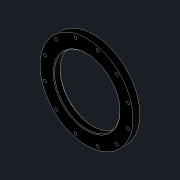
# Autodesk Inventor part: unit-j2-base2
Saved by Autodesk Inventor 2022 (Build 260153000, 153)
## iProperties
Created: 2021-07-12
Part Number: unit-j2-base2
Material: ABS プラスチック
Document SubType Name: Modeling
Designer: yuta0
Density: 1.06 g/cm^3
Appearance: 滑らか - 黒
Mass: 58.1208 g
Surface Area: 198.021 cm^2
Volume: 54.831 cm^3
購入先: 印刷
在庫数: 0.0
Author: yuta0
Autodesk Inventor part; units mm, degrees
ref_plane "YZ Plane" through (0, 0, 0) normal (1, 0, 0) x (0, 1, 0)
ref_plane "XZ Plane" through (0, 0, 0) normal (0, 1, 0) x (-1, 0, 0)
ref_plane "XY Plane" through (0, 0, 0) normal (0, 0, 1) x (1, 0, 0)
sketch "スケッチ1" plane through (0, 0, 0) normal (0, 0, 1) x (1, 0, 0)
  circle A0 centre (0, 0) radius 47.6
  circle A1 centre (0, 0) radius 67.5
  dimension "d0" = 95.2
  dimension "d1" = 135
  constraints: 2 centre point, 2 coincident
  measures "d0" diameter of A0
  measures "d1" diameter of A1
extrude "押し出し1" add sketch "スケッチ1" along normal blind 10
sketch "スケッチ2" plane through (0, 0, 10) normal (0, 0, 1) x (1, 0, 0)
  circle A0 centre (0, 0) radius 62.5
  point P0 (16.1762, 60.3704)
  point P1 (-16.1762, 60.3704)
  point P2 (-44.1942, 44.1942)
  point P3 (-60.3704, 16.1762)
  point P4 (-60.3704, -16.1762)
  point P5 (-44.1942, -44.1942)
  point P6 (-16.1762, -60.3704)
  point P7 (16.1762, -60.3704)
  point P8 (44.1942, -44.1942)
  point P9 (60.3704, -16.1762)
  point P10 (60.3704, 16.1762)
  point P11 (44.1942, 44.1942)
  dimension "d4" = 125
  dimension "d7" = 360
  dimension "d25" = 0
  constraints: 1 coincident, 16 other
  measures "d25" vertical distance of point (-16.176, 60.37) point (16.176, 60.37)
hole "穴1" at (16.1762, 60.3704, 10) at (-16.1762, 60.3704, 10) at (-44.1942, 44.1942, 10) at (-60.3704, 16.1762, 10) at (-60.3704, -16.1762, 10) at (-44.1942, -44.1942, 10) at (-16.1762, -60.3704, 10) at (16.1762, -60.3704, 10) at (44.1942, -44.1942, 10) at (60.3704, -16.1762, 10) at (60.3704, 16.1762, 10) at (44.1942, 44.1942, 10) direction (0, 0, -1) diameter 4.3 end through all clearance for "Flat Head Machine Screw" size "M4" standard "Ansi Metric M Profile"
chamfer "面取り1" distance 1 angle 45 2 edges at (-47.6, 0, 10) (-47.6, 0, 0)
sketch "スケッチ3" plane through (0, 0, 10) normal (0, 0, 1) x (1, 0, 0)
  circle A0 centre (16.1762, 60.3704) radius 2.15 projected
  circle A1 centre (-16.1762, 60.3704) radius 2.15 projected
  circle A2 centre (0, 0) radius 67.5 projected
  circle A3 centre (0, 0) radius 62.5
  circle A4 centre (-16.1762, 60.3704) radius 5
  circle A5 centre (16.1762, 60.3704) radius 5
  point P0 (11.2987, 61.4702)
  point P1 (17.4703, 65.2)
  point P2 (-17.4703, 65.2)
  point P3 (-20.9502, 58.8841)
  constraints: 2 centre point, 2 tangent, 3 other
